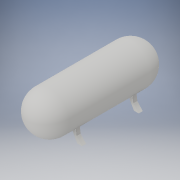
# Autodesk Inventor part: Gascontainer
Saved by Autodesk Inventor 2017 (Build 210142000, 142)
## iProperties
Created: 2017-05-11
Part Number: Gascontainer
Material: Generic
Document SubType Name: Modeling
Designer: Fake
Density: 1 g/cm^3
Appearance: Default
Author: Fake
Autodesk Inventor part; units mm, degrees
ref_plane "YZ Plane" through (0, 0, 0) normal (1, 0, 0) x (0, 1, 0)
ref_plane "XY Plane" through (0, 0, 0) normal (0, 0, 1) x (1, 0, 0)
sketch "Skizze3" plane through (0, 0, 0) normal (1, 0, 0) x (0, 1, 0)
  line L0 (0, 0) -> (1500, 0) construction
  line L1 (0, 0) -> (0, 500)
  line L2 (0, 500) -> (1000, 500)
  line L3 (-320.7107, 0) -> (1924.2641, 0) projected
  line L4 (0, -120.7107) -> (0, 724.2641) projected
  arc A0 (1500, 0) -> (1000, 500) centre (1000, 0) ccw
  line L5 (0, 0) -> (1500, 0)
  dimension "d6" = 1000
  dimension "d7" = 500
  constraints: 8 end point, 2 point on circle, 2 point on line, 1 centre point, 1 collinear, 1 horizontal, 1 line through centre, 1 perpendicular, 1 tangent, 1 vertical
  measures "d6" distance of L1.end L2.end
  measures "d7" distance of L0.start L1.end
revolve "Umdrehung1" add sketch "Skizze3" angle 360 about axis through (0, 0, 0) along (0, 1, 0)
mirror "Spiegeln1" about plane through (0, 0, 500) normal (0, -1, 0) of "Umdrehung1"
ref_plane "Arbeitsebene1" through (0, -750, 0) normal (0, 1, 0) x (-1, 0, 0)
sketch "Skizze4" plane through (0, -750, 0) normal (0, 1, 0) x (-1, 0, 0)
  circle A0 centre (0, 0) radius 500 projected
  circle A1 centre (0, 0) radius 500 projected
  line L0 (-317.8898, -385.9353) -> (-434.1236, -600)
  line L1 (-434.1236, -600) -> (-553.7188, -600)
  line L2 (-553.7188, -600) -> (-419.3789, -449.2772)
  line L3 (-419.3789, -449.2772) -> (-398.8938, -301.4693)
  dimension "d9" = 600
  constraints: 8 end point, 4 point on circle, 1 horizontal
  measures "d9" distance from line of A0.centre L1
extrude "Extrusion2" add sketch "Skizze4" along normal blind 100 contours A0 L0 L1 L2 L3
mirror "Spiegeln2" about plane through (0, 0, 0) normal (1, 0, 0) of "Extrusion2"
mirror "Spiegeln3" about plane through (0, 0, 0) normal (0, 1, 0) of "Extrusion2", "Spiegeln2"
